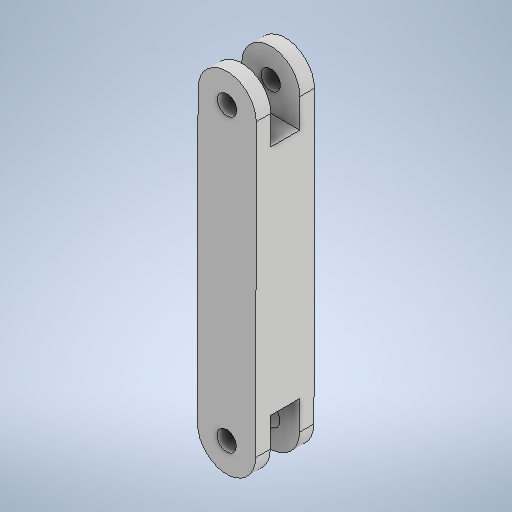
# Autodesk Inventor part: Тяга задняя
Saved by Autodesk Inventor 2025 (Build 290162010, 162A)
## iProperties
Created: 2024-06-14
Part Number: Тяга задняя
Material: Типовые
Document SubType Name: Modeling
Designer: Edward_Higgins
Density: 1 g/cm^3
Appearance: По умолчанию
Author: Edward_Higgins
Autodesk Inventor part; units mm, degrees
ref_plane "YZ Plane" through (0, 0, 0) normal (1, 0, 0) x (0, 1, 0)
ref_plane "XZ Plane" through (0, 0, 0) normal (0, 1, 0) x (-1, 0, 0)
ref_plane "XY Plane" through (0, 0, 0) normal (0, 0, 1) x (1, 0, 0)
sketch "Эскиз1" plane through (0, 0, 0) normal (0, 0, 1) x (1, 0, 0)
  circle A0 centre (0, 0) radius 5
  circle A1 centre (0.2299, 150) radius 5
  line L0 (-14.7701, 150.023) -> (-15, 0.023)
  arc A2 (-15, 0.023) -> (15, -0.023) centre (0, 0) ccw
  line L1 (15, -0.023) -> (15.2299, 149.977)
  arc A3 (15.2299, 149.977) -> (-14.7701, 150.023) centre (0.2299, 150) ccw
  dimension "d0" = 150
  dimension "d1" = 10
  dimension "d2" = 10
  dimension "d3" = 15
  dimension "d4" = 15
  constraints: 4 centre point, 4 end point, 4 point on circle, 4 tangent, 3 coincident
  measures "d0" distance of point (0, 0) A1.centre
  measures "d1" diameter of A0
  measures "d2" diameter of A1
  measures "d3" radius of A3
  measures "d4" radius of A2
extrude "Выдавливание1" add sketch "Эскиз1" along normal mid plane 30
sketch "Эскиз2" plane through (0, 0, 0) normal (1, 0, 0) x (0, 1, 0)
  line L0 (165, -15) -> (165, 15) projected
  line L1 (165, 7.5) -> (135, 7.5)
  line L2 (135, 7.5) -> (135, -7.5)
  line L3 (135, -7.5) -> (165, -7.5)
  line L4 (165, -7.5) -> (165, 7.5)
  line L5 (-15, -15) -> (-15, 15) projected
  line L6 (-15, 7.5) -> (15, 7.5)
  line L7 (15, 7.5) -> (15, -7.5)
  line L8 (15, -7.5) -> (-15, -7.5)
  line L9 (-15, -7.5) -> (-15, 7.5)
  line L10 (145, 15) -> (155, 15) projected
  point P0 (0, 0)
  point P1 (15, 0)
  point P2 (150, 15)
  point P3 (150, 7.5)
  point P4 (0, 7.5)
  dimension "d7" = 15
  constraints: 16 end point, 4 midpoint, 4 parallel, 4 point on line, 3 horizontal alignment, 2 horizontal, 2 perpendicular, 2 vertical alignment
  measures "d7" distance between parallel lines of L1 L3
extrude "Выдавливание2" cut sketch "Эскиз2" along normal mid plane 46.75
